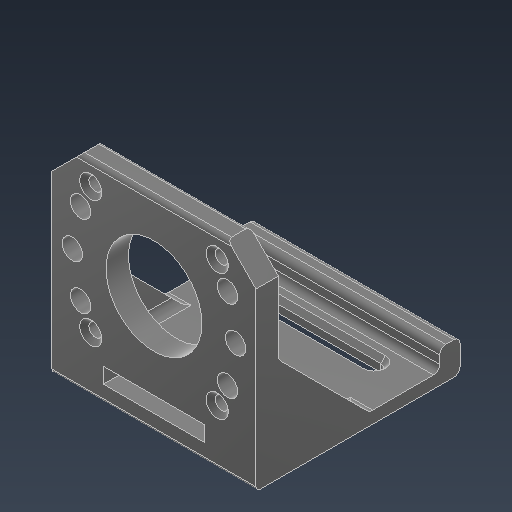
# Autodesk Inventor part: Stepper Mount V4
Saved by Autodesk Inventor 2021.3 (Build 253353000, 353)
## iProperties
Created: 2022-07-20
Part Number: Stepper Mount V4
Material: Thermoplastic Resin
Document SubType Name: Modeling
Designer: david
Density: 1.28 g/cm^3
Appearance: Smooth - Black
Author: david
Autodesk Inventor part; units mm, degrees
ref_plane "YZ Plane" through (0, 0, 0) normal (1, 0, 0) x (0, 1, 0)
ref_plane "XZ Plane" through (0, 0, 0) normal (0, 1, 0) x (-1, 0, 0)
ref_plane "XY Plane" through (0, 0, 0) normal (0, 0, 1) x (1, 0, 0)
sketch "Sketch1" plane through (0, 0, 0) normal (0, 0, 1) x (1, 0, 0)
  line L0 (-21, 21) -> (21, 21)
  line L1 (21, 21) -> (21, -21)
  line L2 (21, -21) -> (-21, -21)
  line L3 (-21, -21) -> (-21, 21)
  line L4 (-21, 21) -> (21, -21) construction
  line L5 (21, 21) -> (-21, -21) construction
  circle A0 centre (15.5, 15.5) radius 1.6
  circle A1 centre (15.5, -15.5) radius 1.6
  line L6 (0, 0) -> (0, 3.2399) construction
  circle A2 centre (-15.5, 15.5) radius 1.6
  circle A3 centre (-15.5, -15.5) radius 1.6
  circle A4 centre (0, 0) radius 11.75
  line L7 (-25, 21) -> (25, 21)
  line L8 (25, 21) -> (25, -26)
  line L9 (25, -26) -> (-25, -26)
  line L10 (-25, -26) -> (-25, 21)
  dimension "d0" = 42
  dimension "d1" = 42
  dimension "d2" = 31
  dimension "d3" = 3.2
  dimension "d4" = 3.2
  dimension "d5" = 23.5
  dimension "d9" = 4
  dimension "d10" = 4
  dimension "d11" = 5
  constraints: 22 end point, 5 centre point, 4 parallel, 2 horizontal, 2 midpoint, 2 perpendicular, 2 point on line, 2 symmetric about line, 1 coincident, 1 vertical, 1 vertical alignment, 2 other
  measures "d0" distance of L0.start L0.end
  measures "d1" distance of L0.end L1.end
  measures "d2" distance of A1.centre A0.centre
  measures "d3" diameter of A0
  measures "d4" diameter of A1
  measures "d5" diameter of A4
  measures "d9" distance of L0.end L7.end
  measures "d10" distance of L7.start L0.start
  measures "d11" distance between parallel lines of L9 L2
extrude "Extrusion1" add sketch "Sketch1" along normal blind 5.5
sketch "Sketch2" plane through (-25, -26, 0) normal (0, -1, 0) x (1, 0, 0)
  line L0 (0, 5.5) -> (50, 5.5) projected
  line L1 (50, 5.5) -> (0, 5.5)
  line L2 (0, 5.5) -> (0, -44.5)
  line L3 (0, -44.5) -> (50, -44.5)
  line L4 (50, -44.5) -> (50, 5.5)
  line L5 (0, 0) -> (0, 5.5) projected
  line L6 (0, 0) -> (50, -44.5) construction
  line L7 (50, 0) -> (0, -44.5) construction
  line L8 (50, 0) -> (0, 0) projected
  line L9 (8.4, -33.5) -> (41.6, -33.5) construction
  line L10 (10, -31.9) -> (40, -31.9)
  line L11 (40, -35.1) -> (10, -35.1)
  arc A0 (10, -31.9) -> (10, -35.1) centre (10, -33.5) ccw
  arc A1 (40, -35.1) -> (40, -31.9) centre (40, -33.5) ccw
  line L12 (8.4, -8.6) -> (41.6, -8.6) construction
  line L13 (10, -7) -> (40, -7)
  line L14 (40, -10.2) -> (10, -10.2)
  arc A2 (10, -7) -> (10, -10.2) centre (10, -8.6) ccw
  arc A3 (40, -10.2) -> (40, -7) centre (40, -8.6) ccw
  point P0 (25, 0)
  point P1 (49.9436, 3)
  point P2 (25, -33.5)
  point P3 (25, -8.6)
  dimension "d12" = 50
  dimension "d71" = 1.6
  dimension "d72" = 1.6
  dimension "d73" = 25
  dimension "d74" = 25
  dimension "d75" = 30
  dimension "d76" = 30
  dimension "d78" = 7
  dimension "d86" = 11
  constraints: 28 end point, 12 point on circle, 8 tangent, 6 point on line, 5 equal length, 4 centre point, 2 horizontal, 2 midpoint, 1 perpendicular
  measures "d12" distance of L0.end L3.end
  measures "d71" radius of A1
  measures "d72" radius of A3
  measures "d73" distance from line of L2 point (25, -33.5)
  measures "d74" distance from line of L2 point (25, -8.6)
  measures "d75" distance of L10.start L10.end
  measures "d76" distance of L14.start L14.end
  measures "d78" distance between parallel lines of L8 L13
  measures "d86" distance from line of L3 A0.centre
extrude "Extrusion2" add sketch "Sketch2" along normal blind 3
sketch "Sketch5" plane through (25, 21, 5.5) normal (1, 0, 0) x (0, 0, -1)
  line L0 (50, -47) -> (5.5, -47) projected
  line L1 (27.75, -47) -> (5.5, -24.75)
  line L2 (5.5, -47) -> (5.5, 0) projected
  point P0 (5.5, -21)
  dimension "d20" = 45
  constraints: 2 end point, 1 midpoint, 1 point on line
  measures "d20" angle of L0 L1
extrude "Extrusion3" add sketch "Sketch5" against normal blind 3.5
mirror "Mirror1" about plane through (0, 0, 0) normal (1, 0, 0) of "Extrusion3"
fillet "Fillet1" radius 2 7 edges at (0, -26, 0) (-21.5, -26, -11.125) (21.5, -26, -11.125) (23.25, -26, -22.25) (23.25, -3.75, 0) (-23.25, -3.75, 0) (-23.25, -26, -22.25)
fillet "Fillet2" radius 0.4 6 edges at (-20.9142, -25.4142, -0.5858) (-21.5, -13.875, 0) (-21.5, -3.3358, 0) (20.9142, -25.4142, -0.5858) (21.5, -3.3358, 0) (21.5, -13.875, 0)
sketch "Sketch6" plane through (-25, -26, 0) normal (0, 1, 0) x (1, 0, 0)
  line L0 (0, -5.5) -> (0, 44.5) projected
  line L1 (50, 44.5) -> (50, -5.5) projected
  line L2 (0, 44.5) -> (50, 44.5)
  line L3 (50, 44.5) -> (50, 39.5)
  line L4 (50, 39.5) -> (0, 39.5)
  line L5 (0, 39.5) -> (0, 44.5)
  point P0 (25, 0)
  point P1 (0, 39.5)
  dimension "d25" = 5
  constraints: 8 end point, 2 parallel, 1 horizontal, 1 perpendicular, 1 point on line
  measures "d25" distance between parallel lines of L2 L4
extrude "Extrusion4" add sketch "Sketch6" along normal blind 5
fillet "Fillet3" radius 1.5 4 edges at (0, -21, -39.5) (0, -21, -44.5) (0, -26, -39.5) (0, -29, -44.5)
sketch "Sketch7" plane through (0, 0, 5.5) normal (0, 0, 1) x (1, 0, 0)
  line L0 (25, 21) -> (-25, 21) projected
  line L1 (-25, 21) -> (-25, -29) projected
  line L2 (25, -29) -> (-25, -29) projected
  line L3 (25, 21) -> (25, -29) projected
  circle A0 centre (15.5, 15.5) radius 1.6 projected
  circle A1 centre (15.5, -15.5) radius 1.6 projected
  circle A2 centre (-15.5, 15.5) radius 1.6 projected
  circle A3 centre (-15.5, -15.5) radius 1.6 projected
  circle A4 centre (0, 0) radius 11.75 projected
  line L4 (35, 0) -> (-35, 0)
  line L5 (0, 0) -> (0, -3.907) construction
  line L6 (-12.4, -24.9) -> (12.4, -24.9)
  line L7 (12.4, -24.9) -> (12.4, -21.1)
  line L8 (12.4, -21.1) -> (-12.4, -21.1)
  line L9 (-12.4, -21.1) -> (-12.4, -24.9)
  line L10 (-12.4, -24.9) -> (12.4, -21.1) construction
  line L11 (12.4, -24.9) -> (-12.4, -21.1) construction
  circle A5 centre (-20, 0) radius 2.5
  circle A6 centre (-18, 10) radius 2.5
  circle A7 centre (-18, -10) radius 2.5
  circle A8 centre (18, -10) radius 2.5
  circle A9 centre (20, 0) radius 2.5
  circle A10 centre (18, 10) radius 2.5
  point P0 (0, -23)
  dimension "d94" = 3.8
  dimension "d95" = 23
  dimension "d96" = 24.8
  dimension "d97" = 12.4
  dimension "d98" = 5
  dimension "d99" = 5
  dimension "d100" = 5
  dimension "d101" = 10
  dimension "d102" = 10
  dimension "d103" = 2
  dimension "d104" = 2
  dimension "d105" = 20
  constraints: 16 end point, 6 centre point, 3 symmetric about line, 2 midpoint, 2 parallel, 1 horizontal, 1 perpendicular, 1 point on line, 1 vertical, 3 other
  measures "d94" distance of L6.end L10.end
  measures "d95" distance of point (0, -23) L5.start
  measures "d96" distance of L6.start L6.end
  measures "d97" distance from line of L7 L5.start
  measures "d98" diameter of A6
  measures "d99" diameter of A5
  measures "d100" diameter of A7
  measures "d101" vertical distance of A5.centre A6.centre
  measures "d102" vertical distance of A5.centre A7.centre
  measures "d103" horizontal distance of A6.centre A5.centre
  measures "d104" horizontal distance of A7.centre A5.centre
  measures "d105" distance of L5.start A5.centre
extrude "Extrusion5" cut sketch "Sketch7" against normal up to surface (5.5 mm away) contours A9 L4 | L4 A9 | A5 L4 | L4 A5 | L9 L8 L7 L6 | A6 | A7 | A8 | A10
sketch "Sketch8" plane through (0, 0, 5.5) normal (0, 0, 1) x (1, 0, 0)
  circle A0 centre (-15.5, 15.5) radius 1.6 projected
  circle A1 centre (15.5, 15.5) radius 1.6 projected
  circle A2 centre (15.5, -15.5) radius 1.6 projected
  circle A3 centre (-15.5, -15.5) radius 1.6 projected
  point P0 (0, 0)
hole "Hole2" at (-15.5, 15.5, 5.5) at (15.5, 15.5, 5.5) at (15.5, -15.5, 5.5) at (-15.5, -15.5, 5.5) direction (0, 0, -1) diameter 3.2 depth 10 countersink diameter 5.45 countersink angle 90
chamfer "Chamfer1" distance 7 angle 45 2 edges at (-25, 21, 2.75) (25, 21, 2.75)
fillet "Fillet4" radius 1 3 edges at (0, -29, 5.5) (0, 21, 5.5) (0, 21, 0)
chamfer "Chamfer2" distance 1.125 angle 45 8 edges at (0, -26, -7) (16.6, -26, -8.6) (0, -26, -10.2) (-16.6, -26, -8.6) (0, -26, -31.9) (16.6, -26, -33.5) (0, -26, -35.1) (-16.6, -26, -33.5)
equation "\"d1\" = d0"
equation "\"d4\" = d3"
equation "\"d10\" = d9"
equation "\"d97\" = 0.5 * d96"
equation "\"d99\" = d98"
equation "\"d100\" = d99"
equation "\"d102\" = d101"
equation "\"d104\" = d103"
body "Solid1"
